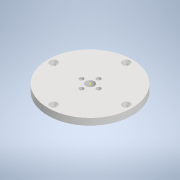
# Autodesk Inventor part: Деталь4
Saved by Autodesk Inventor 2022 (Build 260153000, 153)
## iProperties
Created: 2021-04-19
Part Number: Деталь4
Material: Типовые
Document SubType Name: Sheet Metal
Designer: lbfas
Density: 1 g/cm^3
Appearance: По умолчанию
Sheet Metal Rule: По умолчанию
Author: lbfas
Autodesk Inventor part; units mm, degrees
ref_plane "YZ Plane" through (0, 0, 0) normal (1, 0, 0) x (0, 1, 0)
ref_plane "XZ Plane" through (0, 0, 0) normal (0, 1, 0) x (-1, 0, 0)
sketch "Эскиз1" plane through (0, 0, 0) normal (0, 1, 0) x (-1, 0, 0)
  circle A0 centre (0, 0) radius 44
  circle A1 centre (0, 0) radius 32.5
  dimension "d0" = 88
  dimension "d26" = 65
  constraints: 2 centre point, 2 coincident
  measures "d0" diameter of A0
  measures "d26" diameter of A1
extrude "Выдавливание3" add sketch "Эскиз1" along normal blind 7
sketch "Эскиз20" plane through (0, 7, 0) normal (0, 1, 0) x (1, 0, 0)
  circle A0 centre (38, 0) radius 1.5
  circle A1 centre (0, 38) radius 1.5
  circle A2 centre (-38, 0) radius 1.5
  circle A3 centre (0, -38) radius 1.5
  point P0 (0, 0)
  point P1 (0, 0)
  dimension "d69" = 3
  dimension "d72" = 360
  dimension "d155" = 38
  constraints: 4 centre point, 1 coincident, 9 other
  measures "d69" diameter of A0
  measures "d155" distance of A0.centre point (0, 0)
sketch "Эскиз21" plane through (0, 0, 0) normal (0, -1, 0) x (1, 0, 0)
  circle A0 centre (0, 0) radius 14
  circle A1 centre (0, 0) radius 4.5
  circle A2 centre (-9, 0) radius 2.5
  circle A3 centre (0, -9) radius 2.5
  circle A4 centre (9, 0) radius 2.5
  circle A5 centre (0, 9) radius 2.5
  dimension "d83" = 28
  dimension "d86" = 9
  dimension "d88" = 5
  dimension "d91" = 360
  constraints: 6 centre point, 2 coincident, 9 other
  measures "d83" diameter of A0
  measures "d86" diameter of A1
  measures "d88" diameter of A2
sketch "Эскиз22" plane through (0, 0, 0) normal (0, 1, 0) x (-1, 0, 0)
  circle A0 centre (0, 0) radius 32.5
  constraints: 1 centre point, 1 coincident
extrude "Выдавливание8" add sketch "Эскиз22" along normal blind 3
extrude "Выдавливание10" add sketch "Эскиз21" along normal blind 4.5 contours A0 | A1 | A2 | A3 | A4 | A5
sketch "Эскиз31" plane through (0, 3, 0) normal (0, 1, 0) x (1, 0, 0)
  circle A0 centre (0, 0) radius 32.5
  constraints: 1 centre point, 1 coincident
extrude "Выдавливание15" add sketch "Эскиз31" along normal blind 4
sketch "Эскиз32" plane through (0, 7, 0) normal (0, 1, 0) x (1, 0, 0)
  circle A0 centre (0, 0) radius 4.5
  dimension "d142" = 9
  constraints: 1 centre point, 1 coincident
  measures "d142" diameter of A0
extrude "Выдавливание16" cut sketch "Эскиз32" against normal blind 50
sketch "Эскиз33" plane through (0, 7, 0) normal (0, 1, 0) x (1, 0, 0)
  line L0 (0, 0) -> (9, 0)
  circle A0 centre (9, 0) radius 2.25
  dimension "d145" = 9
  dimension "d146" = 4.5
  constraints: 2 end point, 1 centre point, 1 coincident, 1 horizontal
  measures "d145" distance of L0.start L0.end
  measures "d146" diameter of A0
extrude "Выдавливание17" cut sketch "Эскиз33" against normal blind 9.5
chamfer "Фаска3" distance 2.25 angle 45 1 edges at (6.75, -2.5, 0)
pattern_circular "Круговой массив3" count 4 over 360 about axis through (0, 7, 0) along (0, -1, 0) of "Выдавливание17", "Фаска3"
sketch "Эскиз34" plane through (0, 7, 0) normal (0, 1, 0) x (1, 0, 0)
  point P0 (0, 0)
extrude "Выдавливание18" cut sketch "Эскиз20" against normal blind 10
chamfer "Фаска5" distance 2.5 angle 45 4 edges at (36.5, 7, 0) (-1.5, 7, -38) (-39.5, 7, 0) (-1.5, 7, 38)
ref_plane "РабПлоскость12" through (38, 4.5, 0) normal (-0.6870944, 0, -0.7265681) x (0, -1, 0)
sketch "Эскиз35" plane through (38, 4.5, 0) normal (-0.6870944, 0, -0.7265681) x (0, -1, 0)
  line L0 (0.5774, 1.5) -> (0.5774, 2.5)
  line L1 (0.5774, 2.5) -> (1.1547, 1.5)
  line L2 (0.5774, 1.5) -> (1.1547, 1.5)
  line L3 (0, 1.5) -> (4.5, 1.5) projected
  line L4 (0.5774, 2.5) -> (0, 1.5)
  line L5 (0.5774, 1.5) -> (0, 1.5)
  point P0 (4.5, 27.6096)
  dimension "d164" = 1
  dimension "d165" = 30
  constraints: 10 end point, 1 symmetric about line
  measures "d164" distance of L0.start L0.end
  measures "d165" angle of L0 L1
coil "Пружина2" sketch "Эскиз35" operation cut axis through (38, 4.5, 0) along (0, -1, 0) pitch 1.155 turns 4.329004 hand right
pattern_circular "Круговой массив4" count 4 over 360 about axis through (0, 0, 0) along (0, 1, 0) of "Пружина2"
equation "\"Радиус_гибки\" = Толщина"
equation "\"Ширина_просечки\" = Толщина"
equation "\"Глубина_просечки\" = 0.5 * Толщина"
equation "\"Размер_просечки\" = 4 * Толщина"
equation "\"Мин_остаток\" = 2 * Толщина"
equation "\"Радиус_перехода\" = Радиус_гибки"
equation "\"Радиус_Якоби\" = Радиус_гибки"
equation "\"Размер_зазора\" = Толщина"
equation "\"Толщина\" = 3.048"
